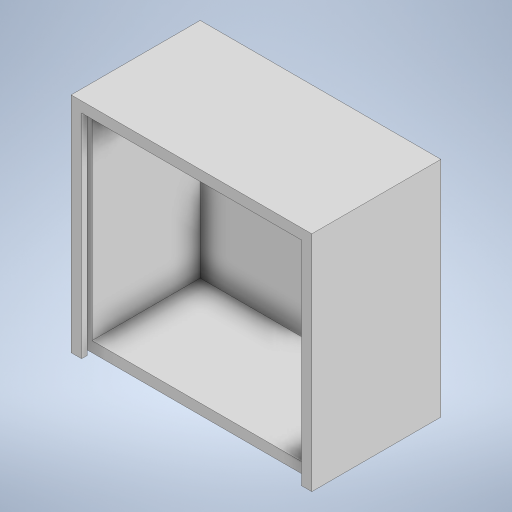
# Autodesk Inventor part: TOP
Saved by Autodesk Inventor 2023 (Build 270158000, 158)
## iProperties
Created: 2024-01-10
Part Number: TOP
Material: Generic
Document SubType Name: Modeling
Designer: magnu
Density: 1 g/cm^3
Appearance: Default
Author: magnu
Autodesk Inventor part; units mm, degrees
ref_plane "YZ Plane" through (0, 0, 0) normal (1, 0, 0) x (0, 1, 0)
ref_plane "XZ Plane" through (0, 0, 0) normal (0, 1, 0) x (-1, 0, 0)
ref_plane "XY Plane" through (0, 0, 0) normal (0, 0, 1) x (1, 0, 0)
sketch "Sketch1" plane through (0, 0, 0) normal (0, 0, 1) x (1, 0, 0)
  line L0 (0, 0) -> (69, 0)
  line L1 (69, 0) -> (69, 64)
  line L2 (69, 64) -> (0, 64)
  line L3 (0, 64) -> (0, 0)
  dimension "d0" = 69
  dimension "d1" = 64
  constraints: 8 end point, 2 parallel, 1 horizontal, 1 perpendicular
  measures "d0" distance of L2.end L1.end
  measures "d1" distance of L1.end L0.end
extrude "Extrusion1" add sketch "Sketch1" along normal blind 37
sketch "Sketch2" plane through (0, 0, 37) normal (0, 0, 1) x (1, 0, 0)
  line L0 (69, 64) -> (0, 64) projected
  line L1 (69, 0) -> (69, 64) projected
  line L2 (0, 64) -> (69, 64)
  line L3 (69, 64) -> (69, 0)
  line L4 (69, 0) -> (0, 0)
  line L5 (0, 0) -> (0, 64)
  line L6 (3, 3) -> (66, 3)
  line L7 (66, 3) -> (66, 61)
  line L8 (66, 61) -> (3, 61)
  line L9 (3, 61) -> (3, 3)
  dimension "d4" = 3
  constraints: 16 end point, 4 parallel, 2 perpendicular, 1 horizontal, 3 other
  measures "d4" distance between parallel lines of L4 L6
extrude "Extrusion2" cut sketch "Sketch2" against normal blind 34 contours L9 L8 L7 L6
sketch "Sketch3" plane through (0, 0, 0) normal (0, -1, 0) x (1, 0, 0)
  line L0 (3, 37) -> (3, 3) projected
  line L1 (66, 37) -> (66, 3) projected
  line L2 (3, 37) -> (66, 37)
  line L3 (66, 37) -> (66, 34)
  line L4 (66, 34) -> (3, 34)
  line L5 (3, 34) -> (3, 37)
  point P0 (0, 0)
  point P1 (3, 34)
  dimension "d7" = 3
  constraints: 8 end point, 2 parallel, 1 horizontal, 1 perpendicular, 1 point on line
  measures "d7" distance of L2.end L3.end
extrude "Extrusion3" cut sketch "Sketch3" against normal up to surface (3 mm away)
sketch "Sketch4" plane through (0, 0, 0) normal (0, -1, 0) x (1, 0, 0)
  line L0 (3, 34) -> (66, 34) projected
  line L1 (34.5, 34) -> (67.5, 34)
  line L2 (67.5, 34) -> (1.5, 34)
  line L3 (1.5, 34) -> (1.5, 35.44)
  line L4 (1.5, 35.44) -> (67.5, 35.44)
  line L5 (67.5, 35.44) -> (67.5, 34)
  point P0 (0, 0)
  dimension "d10" = 33
  dimension "d11" = 66
  dimension "d12" = 1.44
  constraints: 10 end point, 2 parallel, 1 collinear, 1 horizontal, 1 midpoint, 1 perpendicular
  measures "d10" distance of L1.start L1.end
  measures "d11" distance of L3.end L4.end
  measures "d12" distance of L2.end L3.end
extrude "Extrusion4" cut sketch "Sketch4" against normal blind 62.9
body "Solid1"
